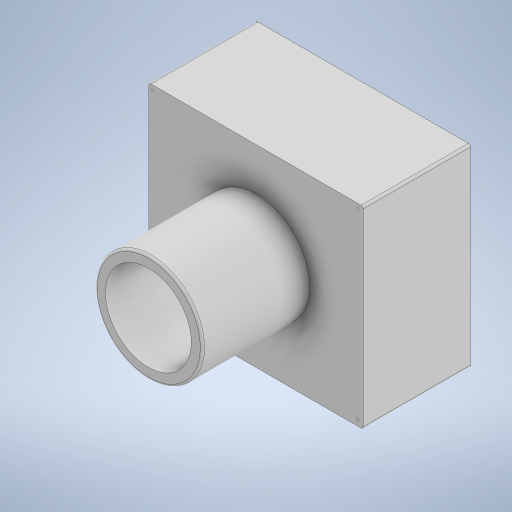
# Autodesk Inventor part: Práctica #1_1104119
Saved by Autodesk Inventor 2024 (Build 280153000, 153)
## iProperties
Created: 2024-02-15
Part Number: Práctica #1_1104119
Material: Genérico
Document SubType Name: Modeling
Designer: ximea
Density: 1 g/cm^3
Appearance: Valor por defecto
Author: ximea
Autodesk Inventor part; units mm, degrees
ref_plane "YZ Plane" through (0, 0, 0) normal (1, 0, 0) x (0, 1, 0)
ref_plane "XZ Plane" through (0, 0, 0) normal (0, 1, 0) x (-1, 0, 0)
ref_plane "XY Plane" through (0, 0, 0) normal (0, 0, 1) x (1, 0, 0)
sketch "Boceto1" plane through (0, 0, 0) normal (0, 0, 1) x (1, 0, 0)
  line L0 (-49, 58.8717) -> (49, 58.8717)
  line L1 (50, 57.8717) -> (50, -30.1283)
  line L2 (49, -31.1283) -> (-49, -31.1283)
  line L3 (-50, -30.1283) -> (-50, 57.8717)
  line L4 (-50, 58.8717) -> (50, -31.1283) construction
  line L5 (50, 58.8717) -> (-50, -31.1283) construction
  circle A0 centre (0, 13.8717) radius 25
  circle A1 centre (0, 13.8717) radius 223
  circle A2 centre (0, 13.8717) radius 23
  arc A3 (-49, 58.8717) -> (-50, 57.8717) centre (-49, 57.8717) ccw
  arc A4 (50, 57.8717) -> (49, 58.8717) centre (49, 57.8717) ccw
  arc A5 (49, -31.1283) -> (50, -30.1283) centre (49, -30.1283) ccw
  arc A6 (-50, -30.1283) -> (-49, -31.1283) centre (-49, -30.1283) ccw
  point P0 (0, 0)
  dimension "d0" = 100
  dimension "d1" = 90
  dimension "d2" = 50
  dimension "d3" = 446
  dimension "d5" = 1
  constraints: 12 end point, 8 point on circle, 8 point on line, 8 tangent, 7 centre point, 3 coincident, 3 equal radius, 2 midpoint, 2 parallel, 1 horizontal, 1 perpendicular
  measures "d0" distance of L4.end L5.end
  measures "d1" distance of L5.start L4.end
  measures "d2" diameter of A0
  measures "d3" diameter of A1
  measures "d5" radius of A3
extrude "Extrusión1" add sketch "Boceto1" against normal blind 50 contours L0 A4 L1 A5 L2 A6 L3 A3
extrude "Extrusión2" add sketch "Boceto1" along normal blind 50 contours A2
extrude "Extrusión3" add sketch "Boceto1" along normal blind 50 contours A0
sketch "Boceto3" plane through (0, 0, 0) normal (0, 0, 1) x (1, 0, 0)
  circle A0 centre (-48.0816, 56.6489) radius 0.5
  circle A1 centre (47.3822, 56.6489) radius 0.5
  circle A2 centre (47.3822, -28.3244) radius 0.5
  circle A3 centre (-48.0816, -28.3244) radius 0.5
  point P0 (0, 0)
  constraints: 4 centre point
extrude "Extrusión4" cut sketch "Boceto3" against normal blind 50 contours A0
extrude "Extrusión5" cut sketch "Boceto3" against normal blind 50 contours A1
extrude "Extrusión6" cut sketch "Boceto3" against normal blind 50 contours A2 | A3
sketch "Boceto4" plane through (0, 13.8717, 50) normal (0, 0, 1) x (1, 0, 0)
  point P0 (0, -13.8717)
  point P1 (-0.1718, 0.0051)
hole "Agujero2" at (-0.1718, 13.8768, 50) direction (0, 0, -1) diameter 40 depth 30
fillet "Empalme1" radius 1 1 edges at (-25, 13.8717, 50)
sketch "Boceto5" plane through (0, 0, 0) normal (0, 0, 1) x (1, 0, 0)
  point P0 (0, 0)
